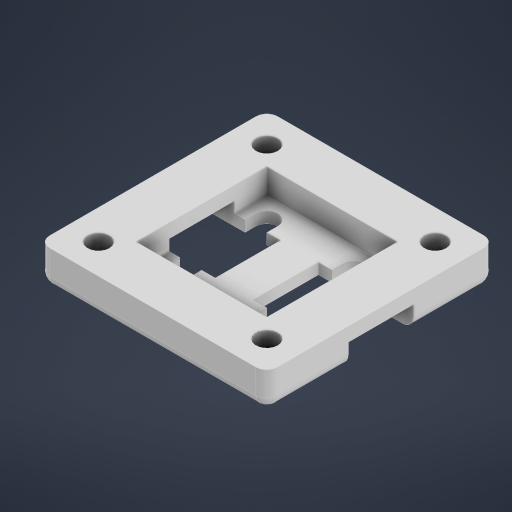
# Autodesk Inventor part: Soporte base PCBs
Saved by Autodesk Inventor 2023 (Build 270158000, 158)
## iProperties
Created: 2021-10-17
Part Number: Soporte base PCBs
Material: Generic
Document SubType Name: Modeling
Designer: jcgg2
Mass: 11.3449 g
Surface Area: 82.1762 cm^2
Volume: 11.3449 cm^3
Density: 1 g/cm^3
Appearance: Default
Author: jcgg2
Autodesk Inventor part; units mm, degrees
ref_plane "YZ Plane" through (0, 0, 0) normal (1, 0, 0) x (0, 1, 0)
ref_plane "XZ Plane" through (0, 0, 0) normal (0, 1, 0) x (-1, 0, 0)
sketch "Sketch1" plane through (0, 0, 0) normal (0, 1, 0) x (-1, 0, 0)
  line L0 (21, 21) -> (-21, 21)
  line L1 (-21, 21) -> (-21, -21)
  line L2 (-21, -21) -> (21, -21)
  line L3 (21, -21) -> (21, 21)
  line L4 (21, 21) -> (-21, -21) construction
  line L5 (-21, 21) -> (21, -21) construction
  point P0 (0, 0)
  dimension "d0" = 42
  dimension "d1" = 42
  constraints: 12 end point, 2 midpoint, 2 parallel, 1 horizontal, 1 perpendicular
  measures "d0" distance of L2.end L1.end
  measures "d1" distance of L1.end L0.end
extrude "Extrusion1" add sketch "Sketch1" along normal blind 6.5
sketch "Sketch2" plane through (0, 6.5, 0) normal (0, 1, 0) x (1, 0, 0)
  line L0 (-12, -12) -> (12, -12)
  line L1 (12, -12) -> (12, 12)
  line L2 (12, 12) -> (-12, 12)
  line L3 (-12, 12) -> (-12, -12)
  line L4 (-12, -12) -> (12, 12) construction
  line L5 (12, -12) -> (-12, 12) construction
  point P0 (0, 0)
  dimension "d4" = 24
  dimension "d5" = 24
  constraints: 12 end point, 2 midpoint, 2 parallel, 1 horizontal, 1 perpendicular
  measures "d4" distance of L2.end L1.end
  measures "d5" distance of L1.end L0.end
extrude "Extrusion2" cut sketch "Sketch2" against normal blind 4.5
sketch "Sketch3" plane through (0, 2, 0) normal (0, 1, 0) x (1, 0, 0)
  line L0 (-10.5, -6) -> (-3.5, -6)
  line L1 (-3.5, -6) -> (-3.5, 6)
  line L2 (-3.5, 6) -> (-10.5, 6)
  line L3 (-10.5, 6) -> (-10.5, -6)
  line L4 (-10.5, -6) -> (-3.5, 6) construction
  line L5 (-3.5, -6) -> (-10.5, 6) construction
  line L6 (-12, -12) -> (-12, 12) projected
  line L7 (3.5, -6) -> (10.5, -6)
  line L8 (10.5, -6) -> (10.5, 6)
  line L9 (10.5, 6) -> (3.5, 6)
  line L10 (3.5, 6) -> (3.5, -6)
  line L11 (3.5, -6) -> (10.5, 6) construction
  line L12 (10.5, -6) -> (3.5, 6) construction
  line L13 (12, 12) -> (12, -12) projected
  point P0 (0, 0)
  point P1 (-7, 0)
  point P2 (-7, 0)
  point P3 (7, 0)
  point P4 (7, 0)
  dimension "d8" = 7
  dimension "d9" = 12
  dimension "d10" = 1.5
  dimension "d11" = 7
  dimension "d12" = 1.5
  dimension "d13" = 12
  constraints: 24 end point, 6 midpoint, 4 parallel, 2 horizontal, 2 horizontal alignment, 2 perpendicular
  measures "d8" distance of L2.end L1.end
  measures "d9" distance of L1.end L0.end
  measures "d10" distance between parallel lines of L6 L3
  measures "d11" distance of L9.end L8.end
  measures "d12" distance between parallel lines of L8 L13
  measures "d13" distance of L7.end L8.end
extrude "Extrusion3" cut sketch "Sketch3" against normal blind 3.5
sketch "Sketch4" plane through (0, 2, 0) normal (0, 1, 0) x (1, 0, 0)
  line L0 (-12, -12) -> (-12, 12) projected
  line L1 (12, -12) -> (-12, -12) projected
  point P0 (0, 0)
  point P1 (-8, -8)
  point P2 (-8, 8)
  point P3 (8, 8)
  point P4 (8, -8)
  dimension "d16" = 16
  dimension "d17" = 16
  dimension "d18" = 4
  dimension "d19" = 4
  constraints: 2 horizontal alignment, 2 vertical alignment
  measures "d16" distance of point (-8, -8) point (-8, 8)
  measures "d17" distance of point (-8, -8) point (8, -8)
  measures "d18" distance from line of L0 point (-8, -8)
  measures "d19" distance from line of L1 point (-8, -8)
hole "Hole1" at (-8, 2, 8) at (-8, 2, -8) at (8, 2, -8) at (8, 2, 8) direction (0, -1, 0) diameter 4 end through all
sketch "Sketch5" plane through (0, 6.5, 0) normal (0, 1, 0) x (1, 0, 0)
  line L0 (-21, -21) -> (21, -21) projected
  line L1 (-21, 21) -> (-21, -21) projected
  point P0 (0, 0)
  point P1 (-15.5, -15.5)
  point P2 (-15.5, 15.5)
  point P3 (15.5, 15.5)
  point P4 (15.5, -15.5)
  dimension "d27" = 31
  dimension "d28" = 31
  dimension "d29" = 5.5
  dimension "d30" = 5.5
  constraints: 2 horizontal alignment, 2 vertical alignment
  measures "d27" distance of point (-15.5, 15.5) point (-15.5, -15.5)
  measures "d28" distance of point (15.5, -15.5) point (-15.5, -15.5)
  measures "d29" distance from line of L0 point (-15.5, -15.5)
  measures "d30" distance from line of L1 point (-15.5, -15.5)
hole "Hole2" at (-15.5, 6.5, 15.5) at (-15.5, 6.5, -15.5) at (15.5, 6.5, -15.5) at (15.5, 6.5, 15.5) direction (0, -1, 0) diameter 4 end through all
sketch "Sketch8" plane through (0, 0, 0) normal (0, -1, 0) x (1, 0, 0)
  line L0 (-21, -21) -> (-21, 21) projected
  line L1 (-21, 21) -> (-25, 21)
  line L2 (-25, 21) -> (-25, -21)
  line L3 (-25, -21) -> (-21, -21)
  line L4 (-21, -21) -> (-21, 21)
  line L5 (21, -21) -> (-21, -21) projected
  point P0 (0, 0)
  point P1 (25, -21)
  dimension "d48" = 4
  constraints: 8 end point, 2 parallel, 1 collinear, 1 horizontal, 1 perpendicular
  measures "d48" distance of L3.end L2.end
extrude "Extrusion6" add sketch "Sketch8" against normal blind 46.5
sketch "Sketch9" plane through (-25, 0, -21) normal (-1, 0, 0) x (0, 0, 1)
  point P0 (21, 0)
ref_plane "Work Plane4" through (25, 0, 21) normal (1, 0, 0) x (0, 0, -1)
sketch "Sketch10" plane through (25, 0, 21) normal (1, 0, 0) x (0, 0, -1)
  line L0 (27, 2) -> (31, 2) projected
  line L1 (27, 2) -> (15, 2) projected
  line L2 (11, 2) -> (15, 2) projected
  line L3 (15, 2) -> (27, 2) projected
  line L4 (27, 2) -> (31, 2) projected
  line L5 (27, 2) -> (15, 2) projected
  line L6 (11, 2) -> (15, 2) projected
  line L7 (15, 2) -> (27, 2) projected
  line L8 (33, 2) -> (9, 2) projected
  line L9 (9, 2) -> (33, 2) projected
  line L10 (27, 2) -> (15, 2) projected
  line L11 (27, 2) -> (27, 0) projected
  line L12 (15, 2) -> (27, 2) projected
  line L13 (15, 2) -> (15, 0) projected
  line L14 (27, 0) -> (15, 0) projected
  point P0 (21, 0)
  constraints: 1 other
extrude "Extrusion7" cut sketch "Sketch10" against normal blind 15
sketch "Sketch11" plane through (-25, 0, -21) normal (-1, 0, 0) x (0, 0, 1)
  line L0 (27, 2) -> (27, 0) projected
  line L1 (15, 2) -> (27, 2) projected
  line L2 (15, 2) -> (15, 0) projected
  line L3 (27, 0) -> (15, 0) projected
  point P0 (21, 0)
extrude "Extrusion8" cut sketch "Sketch11" against normal blind 15
sketch "Sketch12" plane through (-25, 0, 6) normal (-1, 0, 0) x (0, 0, 1)
  line L0 (-27, 0) -> (-27, 46.5) projected
  point P0 (-6, 0)
  point P1 (-21, 41.5)
  point P2 (9, 41.5)
  point P3 (9, 11.5)
  point P4 (-21, 11.5)
  point P5 (-27, 5.5)
  dimension "d55" = 30
  dimension "d56" = 30
  dimension "d57" = 6
  dimension "d92" = 6
  constraints: 2 horizontal alignment, 2 vertical alignment
  measures "d55" distance of point (-21, 11.5) point (-21, 41.5)
  measures "d56" distance of point (9, 11.5) point (-21, 11.5)
  measures "d57" horizontal distance of point (-21, 11.5) point (-27, 5.5)
  measures "d92" distance from line of point (-21, 11.5) L0
hole "Hole3" at (-25, 11.5, -15) at (-25, 11.5, 15) at (-25, 41.5, -15) at (-25, 41.5, 15) direction (1, 0, 0) diameter 3.5 depth 8 tip angle 118
sketch "Sketch13" plane through (-25, 0, 6) normal (-1, 0, 0) x (0, 0, 1)
  circle A0 centre (-21, 41.5) radius 1.75 projected
  circle A1 centre (-21, 11.5) radius 1.75 projected
  circle A2 centre (9, 11.5) radius 1.75 projected
  circle A3 centre (9, 41.5) radius 1.75 projected
  line L0 (0, 2) -> (0, 0) projected
  line L1 (15, 0) -> (0, 0) projected
  line L2 (15, 0) -> (15, 46.5) projected
  line L3 (-27, 46.5) -> (15, 46.5) projected
  line L4 (-27, 0) -> (-27, 46.5) projected
  line L5 (-12, 0) -> (-12, 2) projected
  line L6 (-12, 2) -> (0, 2) projected
  circle A4 centre (-21, 41.5) radius 3.25
  circle A5 centre (9, 41.5) radius 3.25
  circle A6 centre (9, 11.5) radius 3.25
  circle A7 centre (-21, 11.5) radius 3.25
  line L7 (-12, 0) -> (-27, 0) projected
  point P0 (-6, 0)
  dimension "d65" = 1.5
  dimension "d66" = 1.5
  dimension "d67" = 1.5
  dimension "d68" = 1.5
  constraints: 4 centre point
  measures "d65" radial gap between concentric circles of A0 A4
  measures "d66" radial gap between concentric circles of A3 A5
  measures "d67" radial gap between concentric circles of A2 A6
  measures "d68" radial gap between concentric circles of A1 A7
extrude "Extrusion9" add sketch "Sketch13" along normal blind 2 contours A4 | A5 | A6 | A7
fillet "Fillet2" radius 5 2 edges at (-23, 46.5, -21) (-23, 46.5, 21)
fillet "Fillet3" radius 1 4 edges at (-25, 11.5, 11.75) (-25, 41.5, 11.75) (-25, 41.5, -18.25) (-25, 11.5, -18.25)
sketch "Sketch16" plane through (-25, 2, -6) normal (0, -1, 0) x (1, 0, 0)
  line L0 (13, 12) -> (13, 0) projected
  line L1 (0, 12) -> (13, 12) projected
  line L2 (0, 0) -> (0, 12) projected
  line L3 (0, 0) -> (13, 0) projected
  line L4 (37, 0) -> (37, 12) projected
  line L5 (50, 0) -> (37, 0) projected
  line L6 (50, 12) -> (50, 0) projected
  line L7 (50, 12) -> (37, 12) projected
  point P0 (25, 6)
extrude "Extrusion11" cut sketch "Sketch16" against normal blind 2
sketch "Sketch17" plane through (-21, 6.5, 21) normal (1, 0, 0) x (0, 0, -1)
  arc A0 (5, 40) -> (0, 35) centre (5, 35) ccw projected
  line L0 (0, 0) -> (0, 35) projected
  line L1 (42, 0) -> (0, 0) projected
  line L2 (42, 0) -> (42, 35) projected
  arc A1 (42, 35) -> (37, 40) centre (37, 35) ccw projected
  line L3 (5, 40) -> (37, 40) projected
  circle A2 centre (36, 35) radius 1.75 projected
  circle A3 centre (36, 5) radius 1.75 projected
  circle A4 centre (6, 5) radius 1.75 projected
  circle A5 centre (6, 35) radius 1.75 projected
  point P0 (21, -6.5)
extrude "Extrusion12" cut sketch "Sketch17" against normal blind 0.8
sketch "Sketch19" plane through (-25, 0, 6) normal (-1, 0, 0) x (0, 0, 1)
  line L0 (6.5, 18.2831) -> (-6, 11.0662)
  line L1 (-6, 11.0662) -> (-18.5, 18.2831)
  line L2 (-18.5, 18.2831) -> (-18.5, 32.7169)
  line L3 (-18.5, 32.7169) -> (-6, 39.9338)
  line L4 (-6, 39.9338) -> (6.5, 32.7169)
  line L5 (6.5, 32.7169) -> (6.5, 18.2831)
  line L6 (-27, 0) -> (-27, 41.5) projected
  line L7 (-22, 46.5) -> (10, 46.5) projected
  point P0 (-6, 0)
  point P1 (-6, 25.5)
  dimension "d104" = 25
  dimension "d105" = 21
  dimension "d106" = 21
  constraints: 12 end point, 1 vertical, 13 other
  measures "d104" distance between parallel lines of L2 L5
  measures "d105" distance from line of L6 point (-6, 25.5)
  measures "d106" distance from line of L7 point (-6, 25.5)
extrude "Extrusion14" cut sketch "Sketch19" against normal through all
fillet "Fillet4" radius 2 18 edges at (-23.4, 32.7169, -12.5) (-23.4, 39.9338, 0) (-23.4, 18.2831, -12.5) (-23.4, 11.0662, 0) (-23.4, 18.2831, 12.5) (-23.4, 32.7169, 12.5) (-25, 4, 0) (-25, 45.0355, 19.5355) (-25, 46.5, 0) (-25, 45.0355, -19.5355) (-25, 20.75, -21) (-25, 20.75, 21) (21, 0, -13.5) (21, 0, 13.5) (-25, 0, -13.5) (-25, 0, 13.5) (-2, 0, -21) (-2, 0, 21)
sketch "Sketch20" plane through (-21.8, 6.5, 21) normal (1, 0, 0) x (0, 0, -1)
  circle A0 centre (6, 35) radius 2.75
  circle A1 centre (6, 35) radius 1.75 projected
  point P0 (21, -6.5)
  dimension "d110" = 5.5
  constraints: 1 centre point, 1 coincident
  measures "d110" diameter of A0
extrude "Extrusion15" cut sketch "Sketch20" against normal blind 3
pattern_linear "Rectangular Pattern2" count 2 spacing 30 along (0, 0, -1) count 2 spacing 30 along (0, -1, 0) of "Extrusion15"
sketch "Sketch21" plane through (0, 0, 0) normal (0, -1, 0) x (1, 0, 0)
  circle A0 centre (8, 8) radius 2 projected
  circle A1 centre (8, -8) radius 2 projected
  circle A2 centre (-8, -8) radius 2 projected
  circle A3 centre (-8, 8) radius 2 projected
  circle A4 centre (-8, 8) radius 2 projected
  line L0 (-10, 8) -> (-6, 8)
  line L1 (-6, 8) -> (-6, -8)
  line L2 (-6, -8) -> (-10, -8)
  line L3 (-10, -8) -> (-10, 8)
  line L4 (6, 8) -> (10, 8)
  line L5 (10, 8) -> (10, -8)
  line L6 (10, -8) -> (6, -8)
  line L7 (6, -8) -> (6, 8)
  point P0 (0, 0)
  point P1 (8, 6)
  point P2 (8, -6)
  point P3 (-8, -6)
  point P4 (-8, 6)
  point P5 (10, 8)
  point P6 (-6, 8)
  constraints: 16 end point, 4 parallel, 4 point on circle, 2 horizontal, 2 midpoint, 2 perpendicular, 2 point on line, 1 other
extrude "Extrusion16" cut sketch "Sketch21" against normal blind 3 contours L5 A1 L7 A0 | A2 L3 A3 L1
sketch "Sketch22" plane through (-21.8, 6.5, 21) normal (1, 0, 0) x (0, 0, -1)
  circle A0 centre (36, 5) radius 2.75 projected
  circle A1 centre (6, 5) radius 2.75 projected
  circle A2 centre (36, 35) radius 2.75 projected
  circle A3 centre (6, 35) radius 2.75 projected
  line L0 (22, 32.8564) -> (32.5, 26.7942) projected
  arc A4 (33.5, 25.0622) -> (32.5, 26.7942) centre (31.5, 25.0622) ccw projected
  line L1 (33.5, 25.0622) -> (33.5, 12.9378) projected
  arc A5 (32.5, 11.2058) -> (33.5, 12.9378) centre (31.5, 12.9378) ccw projected
  line L2 (32.5, 11.2058) -> (22, 5.1436) projected
  arc A6 (20, 5.1436) -> (22, 5.1436) centre (21, 6.8756) ccw projected
  line L3 (20, 5.1436) -> (9.5, 11.2058) projected
  arc A7 (8.5, 12.9378) -> (9.5, 11.2058) centre (10.5, 12.9378) ccw projected
  line L4 (8.5, 12.9378) -> (8.5, 25.0622) projected
  arc A8 (9.5, 26.7942) -> (8.5, 25.0622) centre (10.5, 25.0622) ccw projected
  line L5 (9.5, 26.7942) -> (20, 32.8564) projected
  arc A9 (22, 32.8564) -> (20, 32.8564) centre (21, 31.1244) ccw projected
  arc A10 (42, 35) -> (37, 40) centre (37, 35) ccw projected
  line L6 (5, 40) -> (37, 40) projected
  arc A11 (5, 40) -> (0, 35) centre (5, 35) ccw projected
  line L7 (0, 0) -> (0, 35) projected
  line L8 (42, 0) -> (0, 0) projected
  line L9 (42, 35) -> (42, 0) projected
  circle A12 centre (36, 35) radius 1.75 projected
  circle A13 centre (36, 5) radius 1.75 projected
  circle A14 centre (6, 5) radius 1.75 projected
  circle A15 centre (6, 35) radius 1.75 projected
  point P0 (21, -6.5)
extrude "Extrusion17" cut sketch "Sketch22" against normal blind 10 contours A0 | A1 | A2 | A3 | L9 L8 L7 A11 L6 A10 | A12 | A13 | A14 | A15
fillet "Fillet5" radius 2 4 edges at (20.4142, 0.5858, 20.4142) (21, 4.25, 21) (20.4142, 0.5858, -20.4142) (21, 4.25, -21)
sketch "Sketch23" plane through (0, 6.5, 0) normal (0, 1, 0) x (1, 0, 0)
  circle A0 centre (15.5, 15.5) radius 2 projected
  circle A1 centre (-15.5, -15.5) radius 2 projected
  circle A2 centre (-15.5, 15.5) radius 2 projected
  circle A3 centre (15.5, -15.5) radius 2 projected
  line L0 (-12, 12) -> (12, 12) projected
  line L1 (12, 12) -> (12, -12) projected
  line L2 (12, -12) -> (-12, -12) projected
  line L3 (-12, -12) -> (-12, 12) projected
  arc A4 (21, 19) -> (19, 21) centre (19, 19) ccw projected
  line L4 (19, 21) -> (-23, 21) projected
  arc A5 (-23, 21) -> (-25, 19) centre (-23, 19) ccw projected
  line L5 (-25, -19) -> (-25, 19) projected
  arc A6 (-25, -19) -> (-23, -21) centre (-23, -19) ccw projected
  line L6 (19, -21) -> (-23, -21) projected
  arc A7 (19, -21) -> (21, -19) centre (19, -19) ccw projected
  line L7 (21, -19) -> (21, 19) projected
  line L8 (0, 0) -> (21, 0)
  line L9 (0, 0) -> (-21, 0)
  line L10 (-21, 0) -> (-21, 21)
  line L11 (-21, 0) -> (-21, -21)
  dimension "d124" = 21
  dimension "d125" = 21
  constraints: 8 end point, 3 point on line, 1 horizontal, 1 midpoint, 1 vertical
  measures "d124" distance of L8.start L8.end
  measures "d125" distance of L8.start L9.end
extrude "Extrusion18" cut sketch "Sketch23" against normal blind 10 contours L11 L6 A6 L5 A5 L4 L10
fillet "Fillet6" radius 2 5 edges at (-21, 0.5858, -20.4142) (-21, 0, -12.5) (-21, 4.25, -21) (-21, 0.5858, 20.4142) (-21, 4.25, 21)
body "Solid1"
